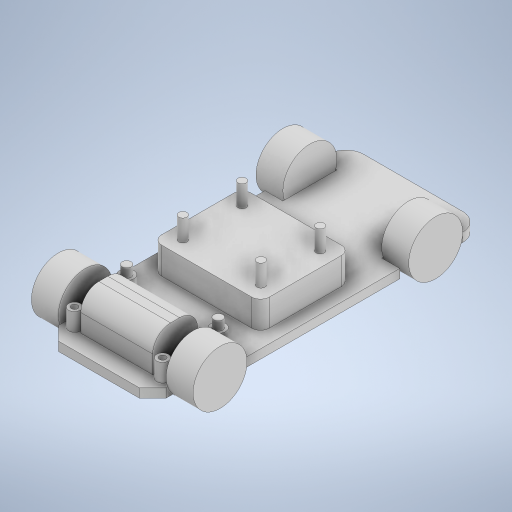
# Autodesk Inventor part: CarApproximation
Saved by Autodesk Inventor 2024.2 (Build 282272000, 272)
## iProperties
Created: 2024-04-01
Part Number: CarApproximation
Material: Generic
Document SubType Name: Modeling
Designer: ringl
Density: 1 g/cm^3
Appearance: Default
Author: ringl
Autodesk Inventor part; units mm, degrees
ref_plane "XZ Plane" through (0, 0, 0) normal (0, 1, 0) x (-1, 0, 0)
ref_plane "XY Plane" through (0, 0, 0) normal (0, 0, 1) x (1, 0, 0)
sketch "Sketch6" plane through (0, 0, 0) normal (0, 1, 0) x (-1, 0, 0)
  line L0 (15, 0) -> (60, 0)
  line L1 (75, -15) -> (75, -165)
  line L2 (65, -175) -> (10, -175)
  line L3 (0, -165) -> (0, -15)
  line L4 (75, -15) -> (60, 0)
  line L5 (15, 0) -> (0, -15)
  arc A0 (65, -175) -> (75, -165) centre (65, -165) ccw
  arc A1 (0, -165) -> (10, -175) centre (10, -165) ccw
  line L6 (7.5, -7.5) -> (7.5, -40)
  line L7 (7.5, -40) -> (0, -40)
  line L8 (67.5, -7.5) -> (67.5, -40)
  line L9 (67.5, -40) -> (75, -40)
  line L10 (75, -160) -> (65, -160)
  line L11 (65, -160) -> (65, -130)
  line L12 (65, -130) -> (75, -130)
  line L13 (75, -130) -> (75, -160)
  line L14 (0, -130) -> (10, -130)
  line L15 (10, -130) -> (10, -160)
  line L16 (10, -160) -> (0, -160)
  line L17 (0, -160) -> (0, -130)
  point P0 (0, 0)
  point P1 (75, -175)
  point P2 (75, 0)
  point P3 (0, -175)
  point P4 (71.25, -40)
  point P5 (70, -160)
  point P6 (0, -160)
  dimension "d30" = 75
  dimension "d31" = 175
  dimension "d32" = 15
  dimension "d33" = 15
  dimension "d34" = 15
  dimension "d35" = 15
  dimension "d36" = 10
  dimension "d37" = 40
  dimension "d38" = 10
  dimension "d39" = 10
  dimension "d40" = 15
  dimension "d41" = 30
  constraints: 36 end point, 16 point on line, 6 parallel, 5 perpendicular, 4 midpoint, 4 point on circle, 4 tangent, 3 horizontal, 2 centre point, 1 equal radius, 1 vertical
  measures "d30" distance of point (75, -175) point (0, -175)
  measures "d31" distance of point (75, 0) point (75, -175)
  measures "d32" distance of L1.start point (75, 0)
  measures "d33" distance of L0.end point (75, 0)
  measures "d34" distance of L0.start point (0, 0)
  measures "d35" distance of L3.end point (0, 0)
  measures "d36" radius of A0
  measures "d37" distance from line of L0 point (71.25, -40)
  measures "d38" distance between parallel lines of L3 L15
  measures "d39" distance between parallel lines of L1 L11
  measures "d40" distance from line of L2 point (70, -160)
  measures "d41" distance between parallel lines of L16 L14
extrude "Extrusion5" add sketch "Sketch6" along normal blind 5 contours L0 L4 L8 L9 L1 L12 L11 L10 A0 L2 A1 L3 L16 L15 L14 L7 L6 L5
sketch "Sketch7" plane through (0, 5, 0) normal (0, 1, 0) x (1, 0, 0)
  line L0 (-67.5, 60) -> (-7.5, 60)
  line L1 (-7.5, 60) -> (-7.5, 110)
  line L2 (-7.5, 110) -> (-67.5, 110)
  line L3 (-67.5, 110) -> (-67.5, 60)
  line L4 (-75, 130) -> (-75, 40) projected
  line L5 (-65, 130) -> (-75, 130) projected
  point P0 (0, 0)
  dimension "d44" = 60
  dimension "d45" = 50
  dimension "d46" = 7.5
  dimension "d47" = 20
  constraints: 8 end point, 2 parallel, 1 horizontal, 1 perpendicular
  measures "d44" distance of L2.end L1.end
  measures "d45" distance of L1.end L0.end
  measures "d46" distance between parallel lines of L4 L3
  measures "d47" distance between parallel lines of L2 L5
extrude "Extrusion6" add sketch "Sketch7" along normal blind 15
sketch "Sketch8" plane through (0, 5, 0) normal (0, 1, 0) x (1, 0, 0)
  line L0 (-57.5, 35) -> (-17.5, 35)
  line L1 (-17.5, 35) -> (-17.5, 10)
  line L2 (-17.5, 10) -> (-57.5, 10)
  line L3 (-57.5, 10) -> (-57.5, 35)
  line L4 (-7.5, 7.5) -> (-7.5, 40) projected
  line L5 (-60, 0) -> (-15, 0) projected
  point P0 (0, 0)
  dimension "d50" = 25
  dimension "d51" = 40
  dimension "d52" = 10
  dimension "d53" = 10
  constraints: 8 end point, 2 parallel, 1 horizontal, 1 perpendicular
  measures "d50" distance of L0.end L1.end
  measures "d51" distance of L0.start L0.end
  measures "d52" distance between parallel lines of L4 L1
  measures "d53" distance between parallel lines of L5 L2
extrude "Extrusion7" add sketch "Sketch8" along normal blind 20
fillet "Fillet2" radius 10 2 edges at (-37.5, 25, -35) (-37.5, 25, -10)
sketch "Sketch9" plane through (-10, 0, -130) normal (1, 0, 0) x (0, 0, -1)
  circle A0 centre (15, 10) radius 15
  line L0 (0, 0) -> (0, 5) projected
  line L1 (0, 0) -> (30, 0) projected
  point P0 (3.8197, 0)
  point P1 (26.1803, 0)
  dimension "d57" = 30
  dimension "d58" = 15
  dimension "d59" = 10
  constraints: 1 centre point
  measures "d57" diameter of A0
  measures "d58" distance from line of L0 A0.centre
  measures "d59" distance from line of L1 A0.centre
extrude "Extrusion8" add sketch "Sketch9" along normal blind 15
ref_plane "Work Plane1" through (-37.5, 0, 0) normal (1, 0, 0) x (0, 1, 0)
mirror "Mirror1" about plane through (-37.5, 0, 0) normal (1, 0, 0) of "Extrusion8"
sketch "Sketch10" plane through (-7.5, 0, -7.5) normal (1, 0, 0) x (0, 0, -1)
  circle A0 centre (15, 10) radius 15
  line L0 (0, 0) -> (0, 5) projected
  line L1 (0, 0) -> (32.5, 0) projected
  point P0 (-7.5, 0)
  point P1 (3.8197, 0)
  point P2 (26.1803, 0)
  dimension "d66" = 30
  dimension "d67" = 15
  dimension "d68" = 10
  constraints: 1 centre point
  measures "d66" diameter of A0
  measures "d67" distance from line of L0 A0.centre
  measures "d68" distance from line of L1 A0.centre
extrude "Extrusion9" add sketch "Sketch10" along normal blind 15
mirror "Mirror2" about plane through (-37.5, 0, 0) normal (1, 0, 0) of "Extrusion9"
fillet "Fillet3" radius 5 4 edges at (-7.5, 12.5, -60) (-7.5, 12.5, -110) (-67.5, 12.5, -110) (-67.5, 12.5, -60)
sketch "Sketch12" plane through (0, 20, 0) normal (0, 1, 0) x (1, 0, 0)
  circle A0 centre (-59.25, 68.5) radius 2.25
  circle A1 centre (-59.25, 101.5) radius 2.25
  circle A2 centre (-15.75, 68.5) radius 2.25
  circle A3 centre (-15.75, 101.5) radius 2.25
  line L0 (-62.5, 60) -> (-12.5, 60) projected
  line L1 (-67.5, 105) -> (-67.5, 65) projected
  point P0 (0, 0)
  dimension "d72" = 4.5
  dimension "d73" = 4.5
  dimension "d74" = 4.5
  dimension "d75" = 4.5
  dimension "d76" = 43.5
  dimension "d77" = 33
  dimension "d78" = 8.5
  dimension "d79" = 8.25
  constraints: 4 centre point, 2 horizontal alignment, 2 vertical alignment
  measures "d72" diameter of A2
  measures "d73" diameter of A3
  measures "d74" diameter of A1
  measures "d75" diameter of A0
  measures "d76" distance of A0.centre A2.centre
  measures "d77" distance of A1.centre A0.centre
  measures "d78" distance from line of L0 A0.centre
  measures "d79" distance from line of L1 A0.centre
extrude "Extrusion10" add sketch "Sketch12" along normal blind 12
sketch "Sketch14" plane through (0, 5, 0) normal (0, 1, 0) x (1, 0, 0)
  circle A0 centre (-63, 41) radius 4
  circle A1 centre (-12, 41) radius 4
  line L0 (0, 40) -> (0, 130) projected
  line L1 (-7.5, 40) -> (0, 40) projected
  circle A2 centre (-62, 11) radius 3.25
  circle A3 centre (-13, 11) radius 3.25
  point P0 (0, 0)
  point P1 (-3.75, 40)
  dimension "d82" = 51
  dimension "d83" = 12
  dimension "d84" = 1
  dimension "d85" = 8
  dimension "d86" = 8
  dimension "d87" = 49
  dimension "d88" = 1
  dimension "d89" = 6.5
  dimension "d90" = 6.5
  dimension "d91" = 30
  constraints: 4 centre point, 2 horizontal alignment, 1 midpoint
  measures "d82" distance of A0.centre A1.centre
  measures "d83" distance from line of L0 A1.centre
  measures "d84" vertical distance of A1.centre point (-3.75, 40)
  measures "d85" diameter of A1
  measures "d86" diameter of A0
  measures "d87" distance of A2.centre A3.centre
  measures "d88" horizontal distance of A0.centre A2.centre
  measures "d89" diameter of A3
  measures "d90" diameter of A2
  measures "d91" vertical distance of A1.centre A3.centre
extrude "Extrusion11" add sketch "Sketch14" along normal blind 5
sketch "Sketch15" plane through (-12, 10, -41) normal (0, 1, 0) x (1, 0, 0)
  circle A0 centre (-51, 0) radius 4 projected
  circle A1 centre (-51, 0) radius 2.5
  circle A2 centre (0, 0) radius 4 projected
  circle A3 centre (0, 0) radius 2.5
  circle A4 centre (-50, -30) radius 3.25 projected
  circle A5 centre (-1, -30) radius 3.25 projected
  circle A6 centre (-51, 0) radius 4
  circle A7 centre (0, 0) radius 4
  circle A8 centre (-1, -30) radius 3.25
  circle A9 centre (-1, -30) radius 1.75
  circle A10 centre (-50, -30) radius 3.25
  circle A11 centre (-50, -30) radius 1.75
  point P0 (12, -41)
  dimension "d94" = 5
  dimension "d95" = 5
  dimension "d96" = 3.5
  dimension "d97" = 3.5
  constraints: 8 centre point, 8 coincident, 4 concentric
  measures "d94" diameter of A1
  measures "d95" diameter of A3
  measures "d96" diameter of A11
  measures "d97" diameter of A9
extrude "Extrusion12" add sketch "Sketch15" along normal blind 5 contours A0 | A1 | A2 | A3 | A4 | A5
sketch "Sketch16" plane through (-63, 15, -41) normal (0, 1, 0) x (1, 0, 0)
  circle A0 centre (0, 0) radius 2.5
  circle A1 centre (51, 0) radius 4 projected
  circle A2 centre (51, 0) radius 2.5
  point P0 (63, -41)
  dimension "d100" = 5
  dimension "d101" = 5
  constraints: 2 centre point, 1 coincident
  measures "d100" diameter of A0
  measures "d101" diameter of A2
extrude "Extrusion13" add sketch "Sketch16" along normal blind 5 contours A0 | A2
equation "\"d33\" = d32"
equation "\"d34\" = d32"
equation "\"d35\" = d34"
body "Solid2"
